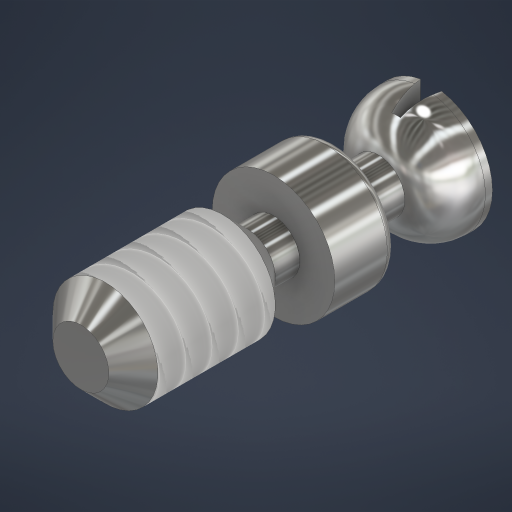
# Autodesk Inventor part: 263.20.150
Saved by Autodesk Inventor 2024 (Build 280153000, 153)
## iProperties
Created: 2023-03-10
Part Number: 263.20.150
Material: Stainless Steel
Document SubType Name: Modeling
Designer: S. Dereskevicius
Density: 8 g/cm^3
Appearance: Semi-Polished
Description: Hafele Rafix S20 Connecting bolt. Drill Hole D5. L=11
Author: sauliusd
Autodesk Inventor part; units mm, degrees
ref_plane "YZ Plane" through (0, 0, 0) normal (1, 0, 0) x (0, 1, 0)
ref_plane "XZ Plane" through (0, 0, 0) normal (0, 1, 0) x (-1, 0, 0)
ref_plane "XY Plane" through (0, 0, 0) normal (0, 0, 1) x (1, 0, 0)
sketch "Sketch1" plane through (0, 0, 0) normal (0, 0, 1) x (1, 0, 0)
  line L0 (-19.8, 0) -> (13.8, 0) projected
  line L1 (0, 0) -> (3.5, 0)
  line L2 (3.5, 0) -> (3.5, 3.5)
  line L3 (3.5, 3.5) -> (0, 3.5)
  line L4 (0, 3.5) -> (0, 0)
  line L5 (3.5, 1.5) -> (6, 1.5)
  arc A0 (8.6, 3.5) -> (6, 1.5) centre (8.6, 0.81) ccw
  line L6 (8.6, 3.5) -> (9, 3.5)
  line L7 (9, 3.5) -> (9, 0)
  line L8 (0, 1.5) -> (-1.5, 1.5)
  line L9 (-1.5, 1.5) -> (-1.5, 0)
  line L10 (-1.5, 0) -> (0, 0)
  line L11 (0, 0) -> (0, 1.5)
  line L12 (-11, 3) -> (-1.5, 3)
  line L13 (-1.5, 3) -> (-1.5, 0)
  line L14 (-1.5, 0) -> (-11, 0)
  line L15 (-11, 0) -> (-11, 3)
  point P0 (-11, 0)
  dimension "d0" = 7
  dimension "d1" = 9
  dimension "d2" = 0.4
  dimension "d18" = 3.5
  dimension "d19" = 3
  dimension "d20" = 2.5
  dimension "d21" = 1.5
  dimension "d22" = 6
  dimension "L" = 11
  constraints: 30 end point, 6 horizontal, 6 parallel, 4 perpendicular, 4 point on line, 3 point on circle, 2 collinear, 1 centre point, 1 coincident, 3 other
  measures "d0" diameter of L3 L0
  measures "d1" distance between parallel lines of L7 L4
  measures "d2" distance of L6.start L6.end
  measures "d18" distance of L2.end L3.end
  measures "d19" diameter of L5 L0
  measures "d20" distance of L5.start L5.end
  measures "d21" distance of L8.start L8.end
  measures "d22" diameter of L12 L0
  measures "L" distance between parallel lines of L4 L15
revolve "Revolution1" add sketch "Sketch1" angle 360 about axis through (-10, 0, 0) along (1, 0, 0)
chamfer "Chamfer1" distance 1.4 angle 45 2 edges at (-1.5, -3, 0) (-11, -3, 0)
fillet "Fillet1" radius 0.5 1 edges at (3.5, -3.5, 0)
sketch "Sketch3" plane through (9, 0, 0) normal (1, 0, 0) x (0, 0, -1)
  line L0 (-3.7, 0.6) -> (3.7, 0.6)
  line L1 (3.7, 0.6) -> (3.7, -0.6)
  line L2 (3.7, -0.6) -> (-3.7, -0.6)
  line L3 (-3.7, -0.6) -> (-3.7, 0.6)
  line L4 (-3.7, 0.6) -> (3.7, -0.6) construction
  line L5 (3.7, 0.6) -> (-3.7, -0.6) construction
  line L6 (-0.6, 2.9) -> (0.6, 2.9)
  line L7 (0.6, 2.9) -> (0.6, -2.9)
  line L8 (0.6, -2.9) -> (-0.6, -2.9)
  line L9 (-0.6, -2.9) -> (-0.6, 2.9)
  line L10 (-0.6, 2.9) -> (0.6, -2.9) construction
  line L11 (0.6, 2.9) -> (-0.6, -2.9) construction
  circle A0 centre (0, 0) radius 3.5 construction
  point P0 (-0.6, 3.448188)
  point P1 (-0.6, 0.6)
  point P2 (-3.448188, 0.6)
  point P3 (-3.448188, -0.6)
  point P4 (-0.6, -0.6)
  point P5 (-0.6, -3.448188)
  point P6 (0.6, -3.448188)
  point P7 (0.6, -0.6)
  point P8 (3.448188, -0.6)
  point P9 (3.448188, 0.6)
  point P10 (0.6, 0.6)
  point P11 (0.6, 3.448188)
  dimension "d28" = 1.2
  dimension "d31" = 0.2
  dimension "d32" = 0.6
  constraints: 24 end point, 4 midpoint, 4 parallel, 3 perpendicular, 2 horizontal
  measures "d28" distance of L0.end L1.end
  measures "d31" distance edge to line of A0 L1
  measures "d32" distance edge to line of A0 L6
sketch "Sketch3 outline for Extrusion1" plane through (9, 0, 0) normal (1, 0, 0) x (0, 0, -1)
  line L0 (-0.6, 0.6) -> (-3.7, 0.6)
  line L1 (-3.7, 0.6) -> (-3.7, -0.6)
  line L2 (-3.7, -0.6) -> (-0.6, -0.6)
  line L3 (-0.6, -0.6) -> (-0.6, -2.9)
  line L4 (-0.6, -2.9) -> (0.6, -2.9)
  line L5 (0.6, -2.9) -> (0.6, -0.6)
  line L6 (0.6, -0.6) -> (3.7, -0.6)
  line L7 (3.7, -0.6) -> (3.7, 0.6)
  line L8 (3.7, 0.6) -> (0.6, 0.6)
  line L9 (0.6, 0.6) -> (0.6, 2.9)
  line L10 (0.6, 2.9) -> (-0.6, 2.9)
  line L11 (-0.6, 2.9) -> (-0.6, 0.6)
extrude "Extrusion1" cut sketch "Sketch3 outline for Extrusion1" against normal blind 2 draft -10
thread "Thread1" size "TR8x1.5" class "7e" standard "ISO Metric Trapezoidal Threads" full length
sketch "Sketch4" plane through (0, 0, 0) normal (0, 0, 1) x (1, 0, 0)
  line L0 (-20.4, 0) -> (3.4, 0) projected
  line L1 (-13, 0) -> (0, 0)
  line L2 (0, 0) -> (0, -2.5)
  line L3 (0, -2.5) -> (-13, -2.5)
  line L4 (-13, -2.5) -> (-13, 0)
  line L5 (0, -3.5) -> (0, 3.5) projected
  line L6 (-11, -1.6) -> (-11, 1.6) projected
  point P0 (0, 0)
  point P1 (0, 0)
  dimension "d36" = 2
  dimension "d37" = 5
  constraints: 8 end point, 2 collinear, 2 parallel, 1 horizontal, 1 perpendicular
  measures "d36" distance between parallel lines of L6 L4
  measures "d37" diameter of L3 L0
revolve "Revolution2" add sketch "Sketch4" angle 360 about axis through (-10, 0, 0) along (1, 0, 0) separate body
